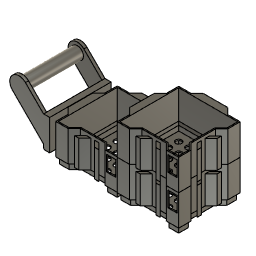
DIY_multipurpose box (Autodesk Fusion 360 design; units mm, degrees)
Autodesk Fusion 360 part; units mm, degrees
sketch "Sketch2" plane through (0, 0, 0) normal (0, 0, 1) x (1, 0, 0)
  line L0 (50, -50) -> (-50, -50)
  line L1 (-50, -50) -> (-50, 50)
  line L2 (-50, 50) -> (50, 50)
  line L3 (50, 50) -> (50, -50)
  line L4 (50, 30) -> (40, 20)
  line L5 (40, 20) -> (40, -20)
  line L6 (40, -20) -> (50, -30)
  line L7 (-30, -50) -> (-20, -40)
  line L8 (-20, -40) -> (20, -40)
  line L9 (20, -40) -> (30, -50)
  line L10 (-50, 29.9) -> (-59.98, 19.92)
  line L11 (-59.98, 19.92) -> (-59.98, -19.92)
  line L12 (-59.98, -19.92) -> (-50, -29.9)
  line L13 (40, 10) -> (50, 20)
  line L14 (40, 3) -> (50, 13)
  line L15 (40, -3) -> (50, -13)
  line L16 (40, -10) -> (50, -20)
  line L17 (-59.98, 10.1) -> (-50, 20.08)
  line L18 (-59.98, 2.9) -> (-50, 12.88)
  line L19 (-59.98, -2.9) -> (-50, -12.88)
  line L20 (-59.98, -10.1) -> (-50, -20.08)
  line L21 (48, 48) -> (48, -48)
  line L22 (48, -48) -> (-48, -48)
  line L23 (-48, -48) -> (-48, 48)
  line L24 (-48, 48) -> (48, 48)
  line L25 (-31.4142, -48.5858) -> (-20.8284, -38)
  line L26 (-20.8284, -38) -> (20.8284, -38)
  line L27 (20.8284, -38) -> (31.4142, -48.5858)
  line L28 (48.5858, 31.4142) -> (38, 20.8284)
  line L29 (38, 20.8284) -> (38, -20.8284)
  line L30 (38, -20.8284) -> (48.5858, -31.4142)
  line L31 (49.8, -19.8) -> (49.8, -12.8)
  line L32 (49.8, 12.8) -> (49.8, 19.8)
  dimension "d9" = 50
  dimension "d10" = 50
  dimension "d11" = 50
  dimension "d12" = 50
  dimension "d13" = 10
  dimension "d14" = 135
  dimension "d15" = 135
  dimension "d16" = 30
  dimension "d17" = 30
  dimension "d18" = 9.98
  dimension "d19" = 135
  dimension "d20" = 135
  dimension "d21" = 3
  dimension "d22" = 3
  dimension "d23" = 10
  dimension "d24" = 10
  dimension "d25" = 29.9
  dimension "d26" = 29.9
  dimension "d27" = 2.9
  dimension "d28" = 10.1
  dimension "d29" = 2.9
  dimension "d30" = 10.1
  dimension "d31" = 10
  dimension "d32" = 135
  dimension "d33" = 135
  dimension "d34" = 30
  dimension "d35" = 30
  dimension "d49" = 2
  dimension "d50" = -2
  dimension "d51" = 2
  dimension "d123" = 49.8
  dimension "d124" = 49.8
  constraint horizontal L0
  constraint perpendicular L0 L1
  constraint parallel L0 L2
  constraint parallel L1 L3
  constraint coincident L3 L4.start
  constraint coincident L3 L6.end
  constraint coincident L0 L7.start
  constraint coincident L0 L9.end
  constraint vertical L5
  constraint horizontal L8
  constraint coincident L1 L10.start
  constraint coincident L1 L12.end
  constraint vertical L11
  constraint coincident L5 L13.start
  constraint coincident L3 L13.end
  constraint coincident L5 L14.start
  constraint coincident L3 L14.end
  constraint parallel L13 L14
  constraint coincident L5 L15.start
  constraint coincident L3 L15.end
  constraint coincident L5 L16.start
  constraint coincident L3 L16.end
  constraint parallel L4 L13
  constraint parallel L6 L15
  constraint parallel L15 L16
  constraint coincident L11 L17.start
  constraint coincident L1 L17.end
  constraint coincident L11 L18.start
  constraint coincident L1 L18.end
  constraint coincident L11 L19.start
  constraint coincident L1 L19.end
  constraint coincident L11 L20.start
  constraint coincident L1 L20.end
  constraint parallel L12 L20
  constraint parallel L12 L19
  constraint parallel L10 L18
  constraint parallel L10 L17
  constraint coincident L16 L31.start
  constraint coincident L15 L31.end
  constraint parallel L3 L31
  constraint coincident L14 L32.start
  constraint coincident L13 L32.end
  constraint parallel L21 L32
  measures "d9" distance of origin L1
  measures "d10" distance of origin L3
  measures "d11" distance of origin L2
  measures "d12" distance of L0 origin
  measures "d13" distance of L3 L5
  measures "d14" angle of L3 L6
  measures "d15" angle of L3 L4
  measures "d16" vertical distance of origin L6.end
  measures "d17" vertical distance of origin L4.start
  measures "d18" distance of L1 L11
  measures "d19" angle of L1 L12
  measures "d20" angle of L1 L10
  measures "d21" vertical distance of origin L15.start
  measures "d22" vertical distance of origin L14.start
  measures "d23" vertical distance of origin L13.start
  measures "d24" vertical distance of origin L16.start
  measures "d25" vertical distance of origin L12.end
  measures "d26" vertical distance of origin L10.start
  measures "d27" vertical distance of origin L18.start
  measures "d28" vertical distance of origin L17.start
  measures "d29" vertical distance of origin L19.start
  measures "d30" vertical distance of origin L20.start
  measures "d31" distance of L0 L8
  measures "d32" angle of L0 L7
  measures "d33" angle of L0 L9
  measures "d34" horizontal distance of origin L7.start
  measures "d35" horizontal distance of origin L9.end
  measures "d123" distance of origin L31
  measures "d124" distance of origin L32
extrude "Extrude2" add sketch "Sketch2" along normal blind 50 contours L0 L3 L6 L9 L21 L22 | L0 L1 L2 L3 L4 L7 L21 L22 L23 L24 | L7 L8 L9 L22 L25 L26 L27 | L4 L5 L6 L21 L28 L29 L30 | L21 L22 L23 L24 L25 L26 L27 L28 L29 L30 makes body 1
extrude "Extrude3" add sketch "Sketch2" along normal blind 45 contours L15 L16 L21 L31 | L5 L15 L16 L21 | L13 L14 L21 L32 | L5 L13 L14 L21 bodies 1
extrude "Extrude4" add sketch "Sketch2" along normal up to surface (50 mm away) contours L1 L11 L12 L20 | L1 L11 L19 L20 | L1 L11 L18 L19 | L1 L11 L17 L18 | L1 L10 L11 L17 bodies 1
extrude "Extrude5" cut sketch "Sketch2" along normal blind 46 contours L1 L11 L19 L20 | L1 L11 L17 L18 bodies 1
extrude "Extrude6" cut sketch "Sketch2" along normal through all contours L21 L22 L23 L24 L25 L26 L27 L28 L29 L30 bodies 1
sketch "Sketch5" plane through (0, -50, 0) normal (0, -1, 0) x (1, 0, 0)
  line L0 (30, 0) -> (50, 0)
  line L1 (50, 0) -> (50, 50)
  line L2 (50, 50) -> (30, 50)
  line L3 (30, 50) -> (30, 0)
  line L4 (47.5, 20) -> (32.5, 20)
  line L5 (32.5, 20) -> (32.5, 45)
  line L6 (32.5, 45) -> (47.5, 45)
  line L7 (47.5, 45) -> (47.5, 20)
  line L8 (47.5, 20) -> (32.5, 45) construction
  line L9 (32.5, 20) -> (47.5, 45) construction
  point P0 (40, 32.5)
  dimension "d149" = 32.5
  dimension "d150" = 47.5
  dimension "d151" = 20
  dimension "d152" = 45
  constraint horizontal L4
  constraint perpendicular L4 L5
  constraint parallel L4 L6
  constraint parallel L5 L7
  constraint coincident L8 P0
  constraint coincident L9 P0
  measures "d149" distance of origin L5
  measures "d150" distance of origin L7
  measures "d151" distance of origin L4
  measures "d152" distance of origin L6
extrude "Extrude13" cut sketch "Sketch5" against normal up to surface (2 mm away) contours L4 L5 L6 L7 bodies 1
pattern_circular "C-Pattern2" count 2 over 270 about axis through (0, 0, 1.75) along (0, 0, 1) of "Extrude3", "Extrude4", "Extrude5"
extrude "Extrude7" add sketch "Sketch2" along normal blind -10 and the other way blind -3 separate body contours L21 L22 L23 L24 L25 L26 L27 L28 L29 L30 makes body 2
sketch "Sketch3" plane through (0, 0, -10) normal (0, 0, -1) x (1, 0, 0)
  line L0 (-20.8284, 38) -> (-30.8284, 48)
  line L1 (-30.8284, 48) -> (-48, 48)
  line L2 (-48, 48) -> (-48, -48)
  line L3 (-48, -48) -> (48, -48)
  line L4 (48, -48) -> (48, -30.8284)
  line L5 (48, -30.8284) -> (38, -20.8284)
  line L6 (38, -20.8284) -> (38, 20.8284)
  line L7 (38, 20.8284) -> (48, 30.8284)
  line L8 (48, 30.8284) -> (48, 48)
  line L9 (48, 48) -> (30.8284, 48)
  line L10 (30.8284, 48) -> (20.8284, 38)
  line L11 (20.8284, 38) -> (-20.8284, 38)
  line L12 (-20.8284, 38) -> (20.8284, 38)
  line L13 (20.8284, 38) -> (31.4142, 48.5858)
  line L14 (38, 20.8284) -> (48.5858, 31.4142)
  line L15 (38, -20.8284) -> (38, 20.8284)
  line L16 (48.5858, -31.4142) -> (38, -20.8284)
  line L17 (-48, -48) -> (48, -48)
  line L18 (-48, 48) -> (-48, -48)
  line L19 (48, -48) -> (48, 48)
  line L20 (-31.4142, 48.5858) -> (-20.8284, 38)
  line L21 (48, 48) -> (-48, 48)
  line L22 (-47, -47) -> (47, -47)
  line L23 (47, -47) -> (47, -31.2426)
  line L24 (47, -31.2426) -> (37, -21.2426)
  line L25 (37, -21.2426) -> (37, 21.2426)
  line L26 (37, 21.2426) -> (47, 31.2426)
  line L27 (47, 31.2426) -> (47, 47)
  line L28 (47, 47) -> (31.2426, 47)
  line L29 (31.2426, 47) -> (21.2426, 37)
  line L30 (21.2426, 37) -> (-21.2426, 37)
  line L31 (-21.2426, 37) -> (-31.2426, 47)
  line L32 (-31.2426, 47) -> (-47, 47)
  line L33 (-47, 47) -> (-47, -47)
  dimension "d55" = -1
extrude "Extrude8" cut sketch "Sketch3" against normal blind 9.5 contours L0 L1 L2 L3 L4 L5 L6 L7 L8 L9 L10 L11 L12 L13 L14 L15 L16 L17 L18 L19 L20 L21 bodies 2
sketch "Sketch4" plane through (0, 0, -10) normal (0, 0, -1) x (1, 0, 0)
  line L0 (-31.2426, 47) -> (-47, 47)
  line L1 (-47, 47) -> (-47, -47)
  line L2 (-47, -47) -> (47, -47)
  line L3 (47, -47) -> (47, -31.2426)
  line L4 (47, -31.2426) -> (37, -21.2426)
  line L5 (37, -21.2426) -> (37, 21.2426)
  line L6 (37, 21.2426) -> (47, 31.2426)
  line L7 (47, 31.2426) -> (47, 47)
  line L8 (47, 47) -> (31.2426, 47)
  line L9 (31.2426, 47) -> (21.2426, 37)
  line L10 (21.2426, 37) -> (-21.2426, 37)
  line L11 (-21.2426, 37) -> (-31.2426, 47)
  line L12 (45, -32.0711) -> (35, -22.0711)
  line L13 (35, -22.0711) -> (35, 22.0711)
  line L14 (35, 22.0711) -> (45, 32.0711)
  line L15 (45, 32.0711) -> (45, 45)
  line L16 (45, 45) -> (32.0711, 45)
  line L17 (32.0711, 45) -> (22.0711, 35)
  line L18 (22.0711, 35) -> (-22.0711, 35)
  line L19 (-22.0711, 35) -> (-32.0711, 45)
  line L20 (-32.0711, 45) -> (-45, 45)
  line L21 (-45, 45) -> (-45, -45)
  line L22 (-45, -45) -> (45, -45)
  line L23 (45, -45) -> (45, -32.0711)
  circle A0 centre (20, -30) radius 5
  circle A1 centre (35, -35) radius 5
  circle A2 centre (35, 35) radius 5
  circle A3 centre (-35, 35) radius 5
  dimension "d60" = -2
  dimension "d64" = 10
  dimension "d65" = 30
  dimension "d66" = 20
  dimension "d73" = 10
  dimension "d74" = 10
  dimension "d75" = 35
  dimension "d76" = 35
  dimension "d77" = 35
  dimension "d78" = 35
  dimension "d81" = 10
  dimension "d82" = 35
  dimension "d83" = 35
  measures "d64" diameter of A0
  measures "d65" vertical distance of origin A0.centre
  measures "d66" horizontal distance of origin A0.centre
  measures "d73" diameter of A1
  measures "d74" diameter of A2
  measures "d75" horizontal distance of origin A2.centre
  measures "d76" vertical distance of origin A2.centre
  measures "d77" vertical distance of origin A1.centre
  measures "d78" horizontal distance of origin A1.centre
  measures "d81" diameter of A3
  measures "d82" vertical distance of origin A3.centre
  measures "d83" horizontal distance of origin A3.centre
extrude "Extrude9" cut sketch "Sketch4" against normal through all contours L12 L13 L14 L15 L16 L17 L18 L19 L20 L21 L22 L23 | A0 | A1 | A2 | A3 bodies 2
extrude "Extrude10" add sketch "Sketch4" against normal blind 2 contours L12 L13 L14 L15 L16 L17 L18 L19 L20 L21 L22 L23 | A0 | A1 | A2 | A3 bodies 2
extrude "Extrude11" cut sketch "Sketch4" along normal through all and the other way through all contours A0 bodies 2
extrude "Extrude12" cut sketch "Sketch4" along normal through all and the other way through all contours A1 | A2 | A3 bodies 2
pattern_linear "R-Pattern1" count 4 spacing 16.6667 along (0, -1, 0) count 4 spacing 16.6667 along (-1, 0, 0) of "Extrude11"
chamfer "Chamfer1" distance 3 angle 45 12 edges at (45, 38.5355, 3) (40, 27.0711, 3) (35, 0, 3) (40, -27.0711, 3) (45, -38.5355, 3) (38.5355, -45, 3) (27.0711, -40, 3) (0, -35, 3) (-27.0711, -40, 3) (-38.5355, -45, 3) (-45, 0, 3) (0, 45, 3) on bodies 2
sketch "Sketch1" plane through (0, 0, 0) normal (0, 1, 0) x (1, 0, 0) in component "handle"
  line L0 (-120, 0) -> (-101, 0)
  line L1 (-101, 0) -> (-101, -44.8)
  line L2 (-101, -44.8) -> (-110, -44.8)
  line L3 (-110, -44.8) -> (-110, -50)
  line L4 (-110, -50) -> (-120, -50)
  line L5 (-120, -7.5736) -> (-120, 0)
  circle A0 centre (-160, -68.7868) radius 15
  circle A1 centre (-160, -68.7868) radius 10
  line L6 (-120, -50) -> (-149.3934, -79.3934)
  line L7 (-120, -7.5736) -> (-170.6066, -58.1802)
  line L8 (-120, -50) -> (-120, -7.5736)
  dimension "d85" = 101
  dimension "d86" = 50
  dimension "d87" = 44.8
  dimension "d88" = 110
  dimension "d89" = 50
  dimension "d90" = 120
  dimension "d91" = 120
  dimension "d93" = 20
  dimension "d94" = 30
  dimension "d95" = 135
  dimension "d96" = 160
  constraint horizontal L0
  constraint vertical L1
  constraint horizontal L2
  constraint vertical L3
  constraint horizontal L4
  constraint vertical L5
  constraint concentric A0 A1
  constraint tangent A0 L6
  constraint tangent A0 L7
  constraint coincident A0 L6.end
  constraint coincident A0 L7.end
  constraint parallel L6 L7
  measures "d85" distance of origin L1
  measures "d86" distance of origin L4
  measures "d87" distance of origin L2
  measures "d88" distance of origin L3
  measures "d89" distance of L0 L4
  measures "d90" distance of origin L5
  measures "d91" horizontal distance of origin L4.end
  measures "d93" diameter of A1
  measures "d94" diameter of A0
  measures "d95" angle of L4 L6
  measures "d96" horizontal distance of origin A0.centre
sketch "Sketch2 (2)" plane through (0, 0, 0) normal (0, 0, 1) x (1, 0, 0) in component "handle"
  line L0 (-100, 50) -> (-110, 50)
  line L1 (-110, 50) -> (-110, -50)
  line L2 (-110, -50) -> (-100, -50)
  line L3 (-100, -50) -> (-100, 50)
  line L4 (-110, -3.1) -> (-100, -13.1)
  line L5 (-110, -9.9) -> (-100, -19.9)
  line L6 (-110, 3.1) -> (-100, 13.1)
  line L7 (-110, 9.9) -> (-100, 19.9)
  dimension "d105" = 100
  dimension "d106" = 110
  dimension "d107" = 50
  dimension "d108" = 50
  dimension "d109" = 45
  dimension "d110" = 45
  dimension "d111" = 3.1
  dimension "d112" = 3.1
  dimension "d113" = 9.9
  dimension "d114" = 9.9
  constraint horizontal L0
  constraint vertical L1
  constraint horizontal L2
  constraint vertical L3
  constraint coincident L1 L4.start
  constraint coincident L3 L4.end
  constraint coincident L1 L5.start
  constraint coincident L3 L5.end
  constraint coincident L1 L6.start
  constraint coincident L3 L6.end
  constraint coincident L1 L7.start
  constraint coincident L3 L7.end
  constraint parallel L4 L5
  constraint parallel L6 L7
  measures "d105" distance of origin L3
  measures "d106" distance of origin L1
  measures "d107" distance of origin L2
  measures "d108" distance of origin L0
  measures "d109" angle of L1 L5
  measures "d110" angle of L1 L7
  measures "d111" vertical distance of origin L4.start
  measures "d112" vertical distance of origin L6.start
  measures "d113" vertical distance of origin L7.start
  measures "d114" vertical distance of origin L5.start
extrude "Extrude1" add sketch "Sketch1" along normal blind 50 and the other way blind 50 separate body contours L0 L1 L2 L3 L4 L5 L8 | A0 L6 L7 L8 | A0 | A1 makes body 3 in component "handle"
extrude "Extrude2'" cut sketch "Sketch1" along normal blind 45 and the other way blind 45 contours A0 L6 L7 L8 | A0 bodies 3 in component "handle"
extrude "Extrude3'" cut sketch "Sketch2 (2)" along normal through all contours L0 L1 L3 L7 | L1 L3 L4 L6 | L1 L2 L3 L5 bodies 3 in component "handle"
fillet "Fillet1" radius 3 1 edges at (-120, 0, 0) on bodies 3 in component "handle"
combine "Combine1" operation add target body 1 tool bodies 2
copy_body "Body->Comp1" bodies 1 removing the originals makes body 4 in component "Box"
component "handle" placed x (1, 0, 0) y (0, 1, 0) z (0, 0, 1) at (0, 0, 0)
component "Box" placed x (1, 0, 0) y (0, 1, 0) z (0, 0, 1) at (-50.02, 0, -0.6)
component "Box" placed x (1, 0, 0) y (0, 1, 0) z (0, 0, 1) at (49.96, 0, -1.1)
component "Box" placed x (1, 0, 0) y (0, 1, 0) z (0, 0, 1) at (49.96, 0, 58.9)
equation "d14 = 90 deg + 45 deg"
equation "d15 = 90 deg + 45 deg"
equation "d19 = 90 deg + 45 deg"
equation "d32 = 90 deg + 45 deg"
equation "d33 = 90 deg + 45 deg"
equation "d48 = 180.0 deg + 90 deg"
equation "d95 = 90 deg + 45 deg"
equation "d150 = d149 + 15 mm"
equation "d152 = d151 + 25 mm"
named bodies: "Box", "handle"
